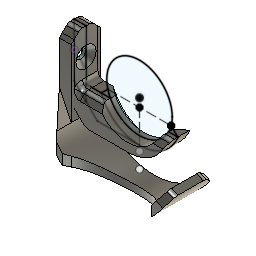
SKADIS_SNS_ToolHooks (Autodesk Fusion 360 design; units mm, degrees)
Autodesk Fusion 360 part; units mm, degrees
sketch "SlotLayout" plane through (0, 0, 0) normal (1, 0, 0) x (0, 1, 0)
  line L0 (-22.4, 25) -> (-22.4, 15)
  line L1 (82.4, 5) -> (82.4, -5)
  line L2 (-37.6, -5) -> (-37.6, 5)
  line L3 (-80, 5) -> (-80, -5) construction
  line L4 (-97.6, 15) -> (-97.6, 25)
  line L5 (2.4, -5) -> (2.4, 5)
  arc A0 (-77.6, 5) -> (-82.4, 5) centre (-80, 5) ccw
  arc A1 (22.4, 25) -> (17.6, 25) centre (20, 25) ccw
  arc A2 (-97.6, 25) -> (-102.4, 25) centre (-100, 25) ccw
  arc A3 (97.6, 15) -> (102.4, 15) centre (100, 15) ccw
  line L6 (-60, 25) -> (-60, 15) construction
  line L7 (-77.6, -5) -> (-77.6, 5)
  arc A4 (77.6, -5) -> (82.4, -5) centre (80, -5) ccw
  line L8 (-40, 5) -> (-40, -5) construction
  line L9 (-57.6, 15) -> (-57.6, 25)
  line L10 (-62.4, 25) -> (-62.4, 15)
  line L11 (-102.4, 25) -> (-102.4, 15)
  line L12 (97.6, 15) -> (97.6, 25)
  arc A5 (-102.4, 15) -> (-97.6, 15) centre (-100, 15) ccw
  line L13 (20, 25) -> (20, 15) construction
  line L14 (22.4, 25) -> (22.4, 15)
  line L15 (-80, 0) -> (0, 0) construction
  line L16 (62.4, 25) -> (62.4, 15)
  line L17 (42.4, 5) -> (42.4, -5)
  arc A6 (2.5, 5) -> (-2.5, 5) centre (0, 5) ccw
  arc A7 (2.4, 5) -> (-2.4, 5) centre (0, 5) ccw
  line L18 (80, 5) -> (80, -5) construction
  arc A8 (82.4, 5) -> (77.6, 5) centre (80, 5) ccw
  arc A9 (-2.5, -5) -> (2.5, -5) centre (0, -5) ccw
  arc A10 (57.6, 15) -> (62.4, 15) centre (60, 15) ccw
  arc A11 (62.4, 25) -> (57.6, 25) centre (60, 25) ccw
  line L19 (17.6, 15) -> (17.6, 25)
  line L20 (-20, 25) -> (-20, 15) construction
  line L21 (-42.4, 5) -> (-42.4, -5)
  line L22 (60, 25) -> (60, 15) construction
  arc A12 (42.4, 5) -> (37.6, 5) centre (40, 5) ccw
  line L23 (-100, 25) -> (-100, 15) construction
  line L24 (100, 25) -> (100, 15) construction
  arc A13 (-57.6, 25) -> (-62.4, 25) centre (-60, 25) ccw
  arc A14 (37.6, -5) -> (42.4, -5) centre (40, -5) ccw
  line L25 (40, 5) -> (40, -5) construction
  line L26 (-17.6, 15) -> (-17.6, 25)
  arc A15 (-17.6, 25) -> (-22.4, 25) centre (-20, 25) ccw
  line L27 (-82.4, 5) -> (-82.4, -5)
  line L28 (-2.5, 5) -> (-2.5, -5)
  line L29 (-2.4, 5) -> (-2.4, -5)
  line L30 (102.4, 25) -> (102.4, 15)
  arc A16 (17.6, 15) -> (22.4, 15) centre (20, 15) ccw
  arc A17 (-22.4, 15) -> (-17.6, 15) centre (-20, 15) ccw
  line L31 (37.6, -5) -> (37.6, 5)
  line L32 (0, 5) -> (0, -5) construction
  arc A18 (-62.4, 15) -> (-57.6, 15) centre (-60, 15) ccw
  arc A19 (-42.4, -5) -> (-37.6, -5) centre (-40, -5) ccw
  arc A20 (-2.4, -5) -> (2.4, -5) centre (0, -5) ccw
  arc A21 (102.4, 25) -> (97.6, 25) centre (100, 25) ccw
  arc A22 (-82.4, -5) -> (-77.6, -5) centre (-80, -5) ccw
  arc A23 (-37.6, 5) -> (-42.4, 5) centre (-40, 5) ccw
  line L33 (77.6, -5) -> (77.6, 5)
  line L34 (57.6, 15) -> (57.6, 25)
  line L35 (2.5, -5) -> (2.5, 5)
  point P0 (-20, 20)
  point P1 (-40, 0)
  dimension "d9" = -40
  dimension "d10" = 0
  dimension "d255" = 0.1
  dimension "d22" = 10
  dimension "d23" = 2.4
  dimension "d4" = 40
  dimension "d25" = 40
  dimension "d26" = 20
  dimension "d27" = 20
  constraint tangent L27 A22
  constraint tangent L7 A22
  constraint parallel L7 L27
  constraint tangent A0 L7
  constraint tangent A0 L27
  constraint vertical L3
  constraint tangent L21 A19
  constraint tangent L2 A19
  constraint parallel L2 L21
  constraint tangent L2 A23
  constraint tangent L21 A23
  constraint vertical L8
  constraint tangent L29 A20
  constraint tangent L5 A20
  constraint parallel L5 L29
  constraint tangent L5 A7
  constraint tangent A7 L29
  constraint parallel L2 L32
  constraint midpoint L15.start L3
  constraint midpoint L15.end L32
  constraint horizontal L15
  constraint equal L8 L32
  constraint equal L3 L8
  constraint midpoint P1 L8
  constraint coincident P1 L15
  constraint equal A7 A23
  constraint equal A0 A23
  constraint coincident L15.end origin
  constraint symmetric A0.end L1.start L32
  constraint symmetric L1.end L27.end L32
  constraint symmetric L7.start A4.start L32
  constraint symmetric A8.end A0.start L32
  constraint symmetric A4 L32 A22
  constraint symmetric A0 A8 L32
  constraint symmetric L17.start L21.start L32
  constraint symmetric L17.end L21.end L32
  constraint symmetric A14.start L2.start L32
  constraint symmetric A12.end L2.end L32
  constraint symmetric A14 L32 A19
  constraint symmetric A12 L32 A23
  constraint tangent L0 A17
  constraint tangent L26 A17
  constraint parallel L0 L26
  constraint tangent L26 A15
  constraint tangent L0 A15
  constraint vertical L20
  constraint equal L20 L32
  constraint equal A7 A15
  constraint midpoint P0 L20
  constraint symmetric L0.end L14.end L32
  constraint symmetric L26.end A1.end L32
  constraint symmetric L0.start A1.start L32
  constraint symmetric L26.start L19.start L32
  constraint symmetric A1 A15 L32
  constraint symmetric A16 A17 L32
  constraint symmetric A11.end L9.end L32
  constraint symmetric L16.start L10.start L32
  constraint symmetric A11 A13 L32
  constraint symmetric L16.end L10.end L32
  constraint symmetric A10.start L9.start L32
  constraint symmetric A10 L32 A18
  constraint symmetric L12.end L4.end L32
  constraint symmetric L30.start A2.end L32
  constraint symmetric A2 L32 A21
  constraint symmetric A3.end L11.end L32
  constraint symmetric A3.start L4.start L32
  constraint symmetric A3 A5 L32
  measures "d22" distance of A6.centre A9.centre
  measures "d23" radius of A7
  measures "d4" distance of L8 L32
  measures "d25" distance of L3 L8
  measures "d26" horizontal distance of L20.end A6.centre
  measures "d27" vertical distance of P0 L15.end
sketch "VerticalPrintKey" plane through (0, 0, 0) normal (1, 0, 0) x (0, 1, 0)
  line L0 (-2.6, 6.7) -> (2.6, 6.7)
  line L1 (2.6, 6.7) -> (2.6, -6.7)
  line L2 (2.6, -6.7) -> (-2.6, -6.7)
  line L3 (-2.6, -6.7) -> (-2.6, 6.7)
  line L4 (0, 6.7) -> (0, -6.7) construction
  circle A0 centre (0, 0) radius 1.6
  line L5 (2.6, 0) -> (20.872204, 0) construction
  line L6 (20.872204, 0) -> (11.736102, 9.136102) construction
  line L7 (11.736102, 9.136102) -> (11.736102, -9.136102) construction
  line L8 (11.736102, -9.136102) -> (20.872204, 0) construction
  dimension "d18" = 13.4
  dimension "d19" = 5.2
  dimension "d20" = 3.2
  constraint horizontal L0
  constraint vertical L1
  constraint horizontal L2
  constraint vertical L3
  constraint midpoint L0 L4.start
  constraint midpoint L2 L4.end
  constraint midpoint L4 A0.centre
  constraint coincident A0.centre origin
  constraint midpoint L1 L5.start
  constraint perpendicular L1 L5
  constraint perpendicular L5 L7
  constraint perpendicular L6 L8
  constraint midpoint L5 L7
  measures "d18" distance of L4.start L4.end
  measures "d19" distance of L1 L3
  measures "d20" diameter of A0
sketch "HorizontalPrintKey" plane through (0, 0, 0) normal (1, 0, 0) x (0, 1, 0)
  circle A0 centre (0, 0) radius 1.6
  line L0 (2.6, -6.7) -> (-2.6, -6.7)
  line L1 (-2.6, -6.7) -> (-2.6, 6.7)
  line L2 (-2.6, 6.7) -> (2.6, 6.7)
  line L3 (2.6, 6.7) -> (2.6, -6.7)
  line L4 (0, 6.7) -> (0, -6.7) construction
  line L5 (0, 6.7) -> (0, 23.593876) construction
  line L6 (0, 23.593876) -> (-8.446938, 15.146938) construction
  line L7 (-8.446938, 15.146938) -> (8.446938, 15.146938) construction
  line L8 (8.446938, 15.146938) -> (0, 23.593876) construction
  line L9 (17.4, -6.7) -> (17.4, 6.7)
  line L10 (17.4, 6.7) -> (22.6, 6.7)
  line L11 (22.6, -6.7) -> (17.4, -6.7)
  line L12 (22.6, 6.7) -> (22.6, -6.7)
  circle A1 centre (20, 0) radius 1.6
  line L13 (37.4, -6.7) -> (37.4, 6.7)
  line L14 (37.4, 6.7) -> (42.6, 6.7)
  line L15 (42.6, -6.7) -> (37.4, -6.7)
  line L16 (42.6, 6.7) -> (42.6, -6.7)
  circle A2 centre (40, 0) radius 1.6
  line L17 (-37.4, 6.7) -> (-42.6, 6.7)
  line L18 (-22.6, -6.7) -> (-17.4, -6.7)
  line L19 (-42.6, -6.7) -> (-37.4, -6.7)
  line L20 (-37.4, -6.7) -> (-37.4, 6.7)
  circle A3 centre (-40, 0) radius 1.6
  circle A4 centre (-20, 0) radius 1.6
  line L21 (-42.6, 6.7) -> (-42.6, -6.7)
  line L22 (-22.6, 6.7) -> (-22.6, -6.7)
  line L23 (-17.4, -6.7) -> (-17.4, 6.7)
  line L24 (-17.4, 6.7) -> (-22.6, 6.7)
  dimension "d21" = 13.4
  dimension "d24" = 5.2
  dimension "d28" = 3.2
  dimension "d32" = 20
  dimension "d33" = 0
  constraint horizontal L2
  constraint vertical L3
  constraint horizontal L0
  constraint vertical L1
  constraint midpoint L4.start L2
  constraint midpoint L4.end L0
  constraint midpoint A0.centre L4
  constraint coincident A0.centre origin
  constraint perpendicular L2 L5
  constraint perpendicular L5 L7
  constraint midpoint L5 L7
  constraint perpendicular L6 L8
  constraint symmetric L5 L9.start L18.end
  constraint symmetric L5 L9.end L23.end
  constraint symmetric L5 L10.end L22.start
  constraint symmetric L5 L11.start L18.start
  constraint symmetric L5 A1 A4
  constraint symmetric L5 L13.start L19.end
  constraint symmetric L5 L13.end L17.start
  constraint symmetric L5 L14.end L17.end
  constraint symmetric L5 L15.start L19.start
  constraint symmetric L5 A2 A3
  measures "d21" distance of L4.end L4.start
  measures "d24" distance of L1 L3
  measures "d28" diameter of A0
sketch "MainProfile" plane through (0, 0, 0) normal (0, 1, 0) x (1, 0, 0) in component "SNS_PSRSelect_Left"
  circle A0 centre (30, 3.786082) radius 22.5 construction
  line L0 (0, -9) -> (0, 9)
  line L1 (0, 9) -> (4, 13)
  line L2 (0, -9) -> (4, -9)
  line L3 (4, -9) -> (4, 13)
  line L4 (0, 0) -> (52.815748, 0) construction
  circle A1 centre (30, 3.786082) radius 26 construction
  arc A2 (45.909903, 19.695985) -> (14.090097, 19.695985) centre (30, 3.786082) ccw
  line L5 (45.909903, 19.695985) -> (51.319805, 14.286082)
  line L6 (4, 9.605887) -> (14.090097, 19.695985)
  line L7 (30, 3.786082) -> (30, 26.286082) construction
  line L8 (4, 13) -> (12.393041, 21.393041)
  arc A3 (47.606959, 21.393041) -> (12.393041, 21.393041) centre (30, 3.786082) ccw
  line L9 (47.606959, 21.393041) -> (53.016861, 15.983139)
  line L10 (0, 9) -> (0, 20.686082)
  line L11 (0, 20.686082) -> (22.752717, 27.608066)
  line L12 (53.016861, 15.983139) -> (51.319805, 14.286082)
  point P0 (30, 28.686082)
  dimension "d34" = 45
  dimension "d35" = 9
  dimension "d37" = 4
  dimension "d38" = 52
  dimension "d41" = 45
  dimension "d42" = 2.4
  dimension "d43" = 30
  dimension "d44" = 12
  dimension "d45" = 9
  dimension "d48" = 8
  constraint vertical L0
  constraint coincident L4.start L0
  constraint perpendicular L0 L2
  constraint perpendicular L2 L3
  constraint coincident L4.start origin
  constraint perpendicular L0 L4
  constraint concentric A0 A1
  constraint parallel L1 L6
  constraint coincident L1.end L3.end
  constraint tangent A2 L6
  constraint tangent A2 L5
  constraint vertical L7
  constraint parallel L1 L8
  constraint tangent L8 A3
  constraint tangent A3 L9
  constraint concentric A2 A3
  constraint parallel L5 L9
  constraint vertical L10
  constraint tangent A3 L11
  constraint perpendicular L5 L12
  measures "d34" diameter of A0
  measures "d35" distance of L4.start L0.start
  measures "d37" distance of L0 L3
  measures "d38" diameter of A1
  measures "d41" angle of L0 L1
  measures "d42" distance of L6 L8
  measures "d43" distance of L0 L7
  measures "d45" distance of L4.start L0.end
extrude "Extrude1" add sketch "MainProfile" along normal mid plane 10 contours L0 L1 L2 L3 | L3 A2 L5 L6 L8 A3 L9 L12 picked at (2.666667, 3.201962) picked at (7.363366, 14.100624) makes body 1 in component "SNS_PSRSelect_Left"
extrude "Extrude2" add sketch "MainProfile" along normal blind 2.4 from surface at -5 contours L1 L8 A3 L10 L11 picked at (5.464347, 18.359708) bodies 1 in component "SNS_PSRSelect_Left"
extrude "Extrude3" cut sketch "HorizontalPrintKey" along normal blind 1.2 contours A0 | L0 L1 L2 L3 picked at (0.595653, -0.335813) picked at (0.039856, -4.998509) bodies 1 in component "SNS_PSRSelect_Left"
extrude "Extrude4" cut sketch "HorizontalPrintKey" along normal blind 8 contours A0 picked at (0.595653, -0.335813) bodies 1 in component "SNS_PSRSelect_Left"
chamfer "Chamfer1" distance 1.8 angle 45 1 edges at (4, -1.491724, 0.578585) on bodies 1 in component "SNS_PSRSelect_Left"
chamfer "Chamfer2" distance 3 angle 45 4 edges at (2, -5, 9) (2, 5, 9) (52.168333, -5, -15.13461) (52.168333, 5, -15.13461) on bodies 1 in component "SNS_PSRSelect_Left"
fillet "Fillet1" radius 2 4 edges at (2, -2, 9) (2, 2, 9) (52.168333, -2, -15.13461) (52.168333, 2, -15.13461) on bodies 1 in component "SNS_PSRSelect_Left"
fillet "Fillet1" radius 10 1 edges at (4, 0, -9.605887) on bodies 1 in component "SNS_PSRSelect_Left"
chamfer "Chamfer3" distance 2 angle 45 2 edges at (6.196521, -2.6, -15.196521) (17.19024, -2.6, -25.138366) on bodies 1 in component "SNS_PSRSelect_Left"
sketch "MainProfile (2)" plane through (0, 0, 0) normal (0, 1, 0) x (1, 0, 0) in component "SNS_PSRSelect_Right"
  circle A0 centre (30, 4) radius 25 construction
  line L0 (0, -9) -> (0, 9)
  line L1 (0, 9) -> (4, 14.673546)
  line L2 (0, -9) -> (4, -9)
  line L3 (4, -9) -> (4, 14.673546)
  line L4 (0, 0) -> (52.815748, 0) construction
  circle A1 centre (30, 4) radius 22.5 construction
  arc A2 (50.432432, 18.405405) -> (9.567568, 18.405405) centre (30, 4) ccw
  line L5 (50.432432, 18.405405) -> (51.42328, 17)
  line L6 (4, 10.508443) -> (9.567568, 18.405405)
  line L7 (30, 4) -> (30, 29) construction
  line L8 (4, 14.673546) -> (7.606054, 19.788324)
  arc A3 (52.393946, 19.788324) -> (7.606054, 19.788324) centre (30, 4) ccw
  line L9 (52.393946, 19.788324) -> (53.384794, 18.382919)
  line L10 (0, 9) -> (0, 23.4)
  line L11 (0, 23.4) -> (21.901758, 30.175914)
  line L12 (53.384794, 18.382919) -> (51.42328, 17)
  point P0 (30, 31.4)
  dimension "d34_1" = 50
  dimension "d35_1" = 9
  dimension "d37_1" = 4
  dimension "d38_1" = 45
  dimension "d42_1" = 2.4
  dimension "d43_1" = 30
  dimension "d44_1" = 12
  dimension "d45_1" = 9
  dimension "d48_1" = 8
  dimension "d73" = 4
  constraint vertical L0
  constraint coincident L4.start L0
  constraint perpendicular L0 L2
  constraint perpendicular L2 L3
  constraint coincident L4.start origin
  constraint perpendicular L0 L4
  constraint concentric A0 A1
  constraint parallel L1 L6
  constraint tangent A2 L6
  constraint tangent A2 L5
  constraint coincident A0.centre A1.centre
  constraint midpoint A2 L7.end
  constraint vertical L7
  constraint parallel L1 L8
  constraint tangent L8 A3
  constraint tangent A3 L9
  constraint concentric A2 A3
  constraint parallel L5 L9
  constraint vertical L10
  constraint tangent A3 L11
  constraint midpoint A3 P0
  constraint perpendicular L5 L12
  measures "d34_1" diameter of A0
  measures "d35_1" distance of L4.start L0.start
  measures "d37_1" distance of L0 L3
  measures "d38_1" diameter of A1
  measures "d42_1" distance of L6 L8
  measures "d43_1" distance of L0 L7
  measures "d45_1" distance of L4.start L0.end
  measures "d48_1" vertical distance of L10.end P0
  measures "d73" distance of L4 A0.centre
extrude "Extrude1'" add sketch "MainProfile (2)" along normal mid plane 10 separate body contours L0 L1 L2 L3 | L3 A2 L5 L6 L8 A3 L9 L12 picked at (2.666667, 3.502814) picked at (5.855856, 14.529131) makes body 2 in component "SNS_PSRSelect_Right"
extrude "Extrude2'" add sketch "MainProfile (2)" against normal blind 2.4 from surface at 5 contours L1 L8 A3 L10 L11 picked at (3.868685, 19.28729) bodies 2 in component "SNS_PSRSelect_Right"
extrude "Extrude5" add sketch "MainProfile (2)" against normal blind 6 from surface at -5 contours L3 A2 L5 L6 L8 A3 L9 L12 picked at (5.855856, 14.529131) bodies 2 in component "SNS_PSRSelect_Right"
sketch "Sketch2" plane through (0, 0, 0) normal (0, 0, 1) x (1, 0, 0) in component "SNS_PSRSelect_Right"
  line L0 (0, 0) -> (52.815748, 0)
  line L1 (30, 0) -> (30, -17.85189) construction
  line L2 (53.384794, -11) -> (53.384794, 5)
  line L3 (13.816779, -11.054397) -> (19.10151, -6.137672)
  line L4 (45.990529, -12.945961) -> (43.2644, -8.904505)
  line L5 (9.567568, -11) -> (4, -11)
  line L6 (4, -5) -> (4, -11)
  line L7 (4, -5) -> (10.817272, -11)
  line L8 (9.567568, -11) -> (50.432432, -11)
  arc A0 (43.2644, -8.904505) -> (19.10151, -6.137672) centre (30, -17.85189) ccw
  point P0 (30, 0)
  point P1 (30, -17.85189)
  point P2 (4, -5)
  point P3 (9.567568, -11)
  point P4 (50.432432, -11)
  point P5 (30, -1.85189)
  dimension "d68" = 3
  dimension "d69" = 32
  constraint coincident L0 P0
  constraint perpendicular L0 L1
  constraint coincident P0 L1.start
  constraint tangent L3 A0
  constraint tangent L4 A0
  constraint coincident P2 L6.start
  measures "d69" diameter of A0
extrude "Extrude6" cut sketch "Sketch2" against normal through all contours L3 L4 L8 A0 | L5 L6 L7 L8 picked at (25.884885, -9.379224) picked at (5.855856, -9) bodies 2 in component "SNS_PSRSelect_Right"
extrude "Extrude3'" cut sketch "HorizontalPrintKey" along normal blind 1.2 contours A0 | L0 L1 L2 L3 picked at (0.595653, -0.335813) picked at (0.039856, -4.998509) bodies 2 in component "SNS_PSRSelect_Right"
extrude "Extrude4'" cut sketch "HorizontalPrintKey" along normal blind 8 contours A0 picked at (0.595653, -0.335813) bodies 2 in component "SNS_PSRSelect_Right"
chamfer "Chamfer1'" distance 1.8 angle 45 1 edges at (4, -1.491724, 0.578585) on bodies 2 in component "SNS_PSRSelect_Right"
chamfer "Chamfer2'" distance 3 angle 45 4 edges at (2, -5, 9) (2, 5, 9) (52.404037, 5, -17.691459) (52.404037, -11, -17.691459) on bodies 2 in component "SNS_PSRSelect_Right"
fillet "Fillet1'" radius 2 4 edges at (2, -2, 9) (2, 2, 9) (52.404037, 2, -17.691459) (52.404037, -8, -17.691459) on bodies 2 in component "SNS_PSRSelect_Right"
fillet "Fillet1'" radius 10 1 edges at (4, 0, -10.508443) on bodies 2 in component "SNS_PSRSelect_Right"
chamfer "Chamfer3'" distance 2 angle 45 2 edges at (3.803027, 2.6, -14.394162) (13.893514, 2.6, -26.166215) on bodies 2 in component "SNS_PSRSelect_Right"
sketch "MainProfile (3)" plane through (0, 0, 0) normal (0, 1, 0) x (1, 0, 0) in component "SNS_HotGlue_01_Left"
  line L0 (0, -9) -> (0, 9)
  line L1 (0, 9) -> (4, 13)
  line L2 (0, -9) -> (4, -9)
  line L3 (4, -9) -> (4, 13)
  line L4 (22, 5.780428) -> (22, 18.555804) construction
  line L5 (4, 13) -> (7.8, 16.8)
  circle A0 centre (22, 3) radius 11
  line L6 (11.357199, 5.780428) -> (32.642801, 5.780428) construction
  line L7 (32.642801, 5.780428) -> (34.862351, 7.999994)
  arc A1 (34.862351, 7.999994) -> (9.137652, 8) centre (22, 3) ccw
  line L8 (22.000003, 16.8) -> (7.8, 16.8)
  line L9 (9.137652, 8) -> (11.357207, 5.780461)
  line L10 (9.137652, 8) -> (12.202041, 8)
  line L11 (34.862351, 7.999994) -> (31.797962, 7.999994)
  line L12 (9.137652, 8) -> (4, 8)
  point P0 (22, 23.792684)
  point P1 (22, 5.780428)
  point P2 (32.642801, 5.780428)
  point P3 (32.642801, 5.780428)
  dimension "d35_2" = 9
  dimension "d37_2" = 4
  dimension "d41_1" = 45
  dimension "d43_2" = 22
  dimension "d45_2" = 9
  dimension "d78" = 22
  dimension "d82" = 2.8
  dimension "d88" = 45.00021
  dimension "d93" = 3
  dimension "d94" = 5
  constraint vertical L0
  constraint coincident origin L0
  constraint perpendicular L0 L2
  constraint perpendicular L2 L3
  constraint coincident L1.end L3.end
  constraint vertical L4
  constraint parallel L1 L5
  constraint perpendicular L4 L6
  constraint coincident L5 L8.end
  constraint tangent A1 L8
  constraint perpendicular L3 L8
  constraint perpendicular L7 L9
  constraint horizontal L10
  constraint parallel L10 L11
  constraint coincident L3 L12.end
  constraint perpendicular L3 L12
  measures "d35_2" distance of origin L0.start
  measures "d37_2" distance of L0 L3
  measures "d41_1" angle of L0 L1
  measures "d43_2" distance of L0 L4
  measures "d45_2" distance of origin L0.end
  measures "d78" diameter of A0
  measures "d82" distance of A0 A1
  measures "d88" angle of L7 L8
  measures "d93" vertical distance of origin A0.centre
  measures "d94" distance of L1.end L12
extrude "Extrude1''" add sketch "MainProfile (3)" along normal mid plane 8 separate body contours L0 L1 L2 L3 | L3 L5 A1 L8 L12 | A0 A1 L10 L11 picked at (1.333333, 2.666667) picked at (7.56998, 13.670943) picked at (21.120076, 15.816) makes body 3 in component "SNS_HotGlue_01_Left"
extrude "Extrude2''" add sketch "MainProfile (3)" against normal blind 2.54 from surface at 4 contours L0 L1 L2 L3 picked at (1.333333, 2.666667) bodies 3 in component "SNS_HotGlue_01_Left"
extrude "Extrude3''" cut sketch "HorizontalPrintKey" along normal blind 1.2 contours A0 | L0 L1 L2 L3 picked at (0.595653, -0.335813) picked at (0.039856, -4.998509) bodies 3 in component "SNS_HotGlue_01_Left"
extrude "Extrude4''" cut sketch "HorizontalPrintKey" along normal blind 8 contours A0 picked at (0.595653, -0.335813) bodies 3 in component "SNS_HotGlue_01_Left"
chamfer "Chamfer1''" distance 1.8 angle 45 1 edges at (4, -1.491724, 0.578585) on bodies 3 in component "SNS_HotGlue_01_Left"
chamfer "Chamfer4" distance 2.8 angle 40 1 edges at (22.000004, 4, -14) measured on face at (6.979217, 4, -10.933333) on bodies 3 in component "SNS_HotGlue_01_Left"
chamfer "Chamfer5" distance 2 angle 45 4 edges at (2, -4, 9) (2, 4, 9) (33.330156, -4, -7.999994) (8.101021, -4, -8) measured on face at (6.979217, -4, -10.933333) measured on face at (7.308209, 4, -11.609506) measured on face at (6.979217, -4, -10.933333) measured on face at (6.979217, -4, -10.933333) on bodies 3 in component "SNS_HotGlue_01_Left"
fillet "Fillet2" radius 2 4 edges at (2, -2, 9) (2, 2, 9) (33.330156, -2, -7.999994) (8.101021, -2, -8) on bodies 3 in component "SNS_HotGlue_01_Left"
fillet "Fillet2" radius 4 1 edges at (7.8, 0, -16.8) on bodies 3 in component "SNS_HotGlue_01_Left"
fillet "Fillet2" radius 2 2 edges at (4, 1, -8) (4, -3, -9) on bodies 3 in component "SNS_HotGlue_01_Left"
sketch "MainProfile (4)" plane through (0, 0, 0) normal (0, 1, 0) x (1, 0, 0) in component "SNS_HotGlue_01_Right"
  circle A0 centre (22, 8) radius 20 construction
  line L0 (0, -9) -> (0, 13)
  line L1 (0, 13) -> (4, 21.332667)
  line L2 (0, -9) -> (4, -9)
  line L3 (4, -9) -> (4, 16.717798)
  line L4 (0, 0) -> (52.815748, 0) construction
  arc A1 (40, 16.717798) -> (4, 16.717798) centre (22, 8) ccw
  line L5 (22, 3) -> (22, 28) construction
  line L6 (0, 13) -> (0, 22.059554)
  line L7 (0, 22.059554) -> (12.003271, 28.045583)
  line L8 (22, 5.780428) -> (22, 18.555804)
  arc A2 (42.243399, 17.589828) -> (4, 21.332667) centre (22, 8) ccw
  line L9 (40, 16.717798) -> (42.243399, 17.589828)
  line L10 (4, 16.717798) -> (4, 21.332667)
  line L11 (4, 16.717798) -> (0, 8.385131)
  point P0 (22, 3)
  dimension "d34_1_1" = 40
  dimension "d35_1_1" = 9
  dimension "d37_1_1" = 4
  dimension "d45_1_1" = 13
  dimension "d105" = 25
  dimension "d106" = 2.4
  constraint vertical L0
  constraint coincident L4.start L0
  constraint perpendicular L0 L2
  constraint perpendicular L2 L3
  constraint coincident L4.start origin
  constraint perpendicular L0 L4
  constraint coincident A0.centre A1.centre
  constraint midpoint A1 L5.end
  constraint vertical L5
  constraint vertical L6
  constraint coincident P0 L5.start
  constraint coincident A0.centre L5
  constraint tangent L7 A2
  constraint vertical L10
  constraint parallel L1 L11
  measures "d34_1_1" diameter of A0
  measures "d35_1_1" distance of L4.start L0.start
  measures "d37_1_1" distance of L0 L3
  measures "d45_1_1" distance of L4.start L0.end
  measures "d105" distance of P0 L5.end
  measures "d106" distance of A1 A2
extrude "Extrude1'''" add sketch "MainProfile (4)" along normal mid plane 10 separate body contours L0 L2 L3 L11 | L0 L1 L10 L11 | A1 A2 L9 L10 picked at (2.666667, 5.367643) picked at (2.666667, 17.016822) picked at (13.902381, 27.981868) makes body 4 in component "SNS_HotGlue_01_Right"
extrude "Extrude2'''" add sketch "MainProfile (4)" against normal blind 2.4 from surface at 5 contours L1 L6 L7 A2 picked at (1.333333, 18.797407) bodies 4 in component "SNS_HotGlue_01_Right"
extrude "Extrude5'" add sketch "MainProfile (4)" against normal blind 6 from surface at -5 contours L0 L1 L10 L11 | A1 A2 L9 L10 picked at (2.666667, 17.016822) picked at (13.902381, 27.981868) bodies 4 in component "SNS_HotGlue_01_Right"
sketch "Sketch2 (2)" plane through (0, 0, 0) normal (0, 0, 1) x (1, 0, 0) in component "SNS_HotGlue_01_Right"
  line L0 (0, 0) -> (52.815748, 0)
  line L1 (22, 0) -> (22, -17) construction
  line L2 (37, -11) -> (35.890182, -9.058788)
  line L3 (7, -11) -> (37, -11)
  arc A0 (35.890182, -9.058788) -> (8.109818, -9.058788) centre (22, -17) ccw
  line L4 (8.109818, -9.058788) -> (7, -11)
  line L5 (0, -5) -> (5, -11)
  line L6 (5, -11) -> (0, -11)
  line L7 (0, -11) -> (0, -5)
  point P0 (22, -17)
  point P1 (22, -1)
  point P2 (40, -11)
  point P3 (4, -5)
  point P4 (4, -11)
  point P5 (0, -5)
  dimension "d69_1" = 32
  dimension "d107" = 30
  dimension "d108" = 6
  dimension "d109" = 2
  constraint coincident L0 L1.start
  constraint perpendicular L0 L1
  constraint coincident P0 L1.end
  constraint coincident L1 P0
  constraint tangent L2 A0
  constraint coincident L1 P1
  constraint coincident P1 A0
  constraint coincident L3 L2.start
  constraint coincident L3 L4.end
  constraint tangent A0 L4
  constraint coincident L3.start L4.end
  constraint horizontal L2.start P2
  constraint horizontal L3
  constraint coincident P5 L5.start
  constraint parallel L3 L6
  constraint perpendicular L3 L7
  constraint horizontal P4 L5.end
  measures "d69_1" diameter of A0
  measures "d107" distance of L3.start L2.start
  measures "d108" distance of P0 L3
  measures "d109" distance of L3.start L5.end
extrude "Extrude6'" cut sketch "Sketch2 (2)" against normal through all contours L2 L3 A0 L4 | L5 L6 L7 picked at (24.01515, -5.202888) picked at (1.666667, -9) bodies 4 in component "SNS_HotGlue_01_Right"
extrude "Extrude3'''" cut sketch "HorizontalPrintKey" along normal blind 1.2 contours A0 | L0 L1 L2 L3 picked at (0.595653, -0.335813) picked at (0.039856, -4.998509) bodies 4 in component "SNS_HotGlue_01_Right"
extrude "Extrude4'''" cut sketch "HorizontalPrintKey" along normal blind 8 contours A0 picked at (0.595653, -0.335813) bodies 4 in component "SNS_HotGlue_01_Right"
chamfer "Chamfer1'''" distance 1.8 angle 45 1 edges at (4, -1.491724, 0.578585) on bodies 4 in component "SNS_HotGlue_01_Right"
chamfer "Chamfer2''" distance 3 angle 45 4 edges at (2, 5, 9) (41.121699, 5, -17.153813) (41.121699, -11, -17.153813) (2, -5, 9) on bodies 4 in component "SNS_HotGlue_01_Right"
fillet "Fillet1''" radius 2 4 edges at (2, 2, 9) (41.121699, -8, -17.153813) (41.121699, 2, -17.153813) (2, -2, 9) on bodies 4 in component "SNS_HotGlue_01_Right"
chamfer "Chamfer3''" distance 1 angle 45 2 edges at (2, 2.6, -17.166333) (7.604861, 2.6, -25.162167) on bodies 4 in component "SNS_HotGlue_01_Right"
component "SNS_PSRSelect" placed x (1, 0, 0) y (0, 1, 0) z (0, 0, 1) at (0, 0, 0)
component "SNS_HotGlueGun_01" placed x (1, 0, 0) y (0, 1, 0) z (0, 0, 1) at (0, 0, 0)
component "SNS_PSRSelect_Right" placed x (1, 0, 0) y (0, 1, 0) z (0, 0, 1) at (0, 0, 0) in component "SNS_PSRSelect"
component "SNS_PSRSelect_Left" placed x (1, 0, 0) y (0, 1, 0) z (0, 0, 1) at (0, 0, 0) in component "SNS_PSRSelect"
component "SNS_HotGlue_01_Left" placed x (1, 0, 0) y (0, 1, 0) z (0, 0, 1) at (0, 0, 0) in component "SNS_HotGlueGun_01"
component "SNS_HotGlue_01_Right" placed x (1, 0, 0) y (0, 1, 0) z (0, 0, 1) at (0, 0, 0) in component "SNS_HotGlueGun_01"
equation "XY_Tolerance = 0.2 mm"
equation "Z_Tolerance = 0.2 mm"
equation "Wall_Thickness = 0.4 mm"
equation "Layer_Height = 0.2 mm"
equation "M3Hole_wClearance = 3.2 mm"
equation "M3Hole_wSelfTapping = 2.8 mm"
equation "d20 = M3Hole_wClearance"
equation "d28 = M3Hole_wClearance"
equation "M3Hole_CounterSink = 1.8 mm"
equation "d56 = M3Hole_CounterSink"
equation "d56_1 = M3Hole_CounterSink"
equation "d56_2 = M3Hole_CounterSink"
equation "d56_1_1 = M3Hole_CounterSink"
named bodies: "PSRSelect_Left", "PSRSelect_Right", "HotGlue_01_Left", "HotGlue_01_Right"
